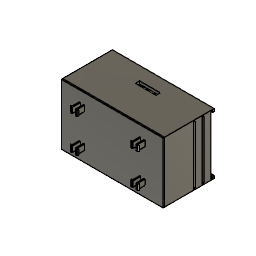
Control board - base v9 (Autodesk Fusion 360 design; units mm, degrees)
Autodesk Fusion 360 part; units mm, degrees
note: some values were not read from the file. Chosen so that the rebuilt part matches the saved one: which bodies a step acts on.
sketch "Esquisse1" plane through (0, 0, 0) normal (0, 1, 0) x (1, 0, 0)
  line L0 (-11.4317, -0.2961) -> (62.5683, -0.2961)
  line L1 (62.5683, -0.2961) -> (62.5683, -44.2961)
  line L2 (62.5683, -44.2961) -> (-11.4317, -44.2961)
  line L3 (-11.4317, -44.2961) -> (-11.4317, -0.2961)
  dimension "d1" = 74
  dimension "d2" = 44
  constraint horizontal L0
  constraint vertical L1
  constraint horizontal L2
  constraint vertical L3
  measures "d1" distance of L1 L3
  measures "d2" distance of L0 L2
extrude "Extrusion1" add sketch "Esquisse1" along normal blind 37.2 makes body 1
shell "Coque1" thickness 2 removed faces 1 at (37.9017, 37.2, 29.6294) on bodies 1
sketch "Sketch4" plane through (62.5683, 0, 0) normal (1, 0, 0) x (0, 1, 0)
  line L0 (0, 44.2961) -> (0, 0.2961)
  line L1 (0, 0.2961) -> (37.2, 0.2961)
  line L2 (37.2, 0.2961) -> (37.2, 44.2961)
  line L3 (37.2, 44.2961) -> (0, 44.2961)
  line L4 (0, 22.2961) -> (37.2, 22.2961) construction
  line L5 (22, 43.3961) -> (23.4, 43.3961)
  line L6 (23.4, 43.3961) -> (23.4, 1.1961)
  line L7 (23.4, 1.1961) -> (22, 1.1961)
  line L8 (22, 1.1961) -> (22, 43.3961)
  line L9 (29.8, 1.1961) -> (28.4, 1.1961)
  line L10 (28.4, 1.1961) -> (28.4, 43.3961)
  line L11 (28.4, 43.3961) -> (29.8, 43.3961)
  line L12 (29.8, 43.3961) -> (29.8, 1.1961)
  line L13 (34.8, 43.3961) -> (36.2, 43.3961)
  line L14 (36.2, 43.3961) -> (36.2, 1.1961)
  line L15 (36.2, 1.1961) -> (34.8, 1.1961)
  line L16 (34.8, 1.1961) -> (34.8, 43.3961)
  line L17 (36.2, 2.2961) -> (37.2, 2.2961)
  line L18 (37.2, 2.2961) -> (37.2, 42.2961)
  line L19 (37.2, 42.2961) -> (36.2, 42.2961)
  line L20 (36.2, 42.2961) -> (36.2, 2.2961)
  dimension "d16" = 42.2
  dimension "d17" = 42.2
  dimension "d18" = 42.2
  dimension "d19" = 1.4
  dimension "d20" = 1.4
  dimension "d21" = 1.4
  dimension "d54" = 22
  dimension "d55" = 5
  dimension "d56" = 5
  dimension "d57" = 40
  constraint midpoint L0 L4.start
  constraint midpoint L2 L4.end
  constraint horizontal L5
  constraint vertical L6
  constraint horizontal L7
  constraint vertical L8
  constraint symmetric L4 L5 L7
  constraint horizontal L9
  constraint vertical L10
  constraint horizontal L11
  constraint vertical L12
  constraint horizontal L13
  constraint vertical L14
  constraint horizontal L15
  constraint vertical L16
  constraint symmetric L4 L9 L11
  constraint symmetric L4 L13 L15
  constraint horizontal L17
  constraint vertical L18
  constraint horizontal L19
  constraint vertical L20
  constraint coincident L2 L18.end
  constraint coincident L14 L17.start
  constraint symmetric L4 L17 L19
  measures "d16" distance of L5.start L7.end
  measures "d17" distance of L9.end L10.end
  measures "d18" distance of L13.start L15.end
  measures "d19" distance of L6.end L7.end
  measures "d20" distance of L9.start L9.end
  measures "d21" distance of L14.end L15.end
  measures "d54" distance of L0 L8
  measures "d55" distance of L6 L10
  measures "d56" distance of L12 L16
  measures "d57" distance of L17.end L18.end
extrude "Extrude4" cut sketch "Sketch4" against normal blind 73.1 contours L13 L14 L15 L16 L20 | L5 L6 L7 L8 | L9 L10 L11 L12 bodies 1
ref_plane "WorkPlane1" through (25.5683, 18.6, 32.4961) normal (0, 0, 1) x (1, 0, 0)
sketch "Sketch5" plane through (0, 0, 32.4961) normal (0, 0, 1) x (1, 0, 0)
  line L0 (2.3683, 0) -> (2.3683, -5.74)
  line L1 (2.1083, -6) -> (1.3083, -6)
  line L2 (1.1018, -5.8979) -> (0.5683, -5.2)
  line L3 (0.5683, -5.2) -> (1.5683, -5.2)
  line L4 (1.5683, -5.2) -> (1.5683, 0)
  line L5 (1.5683, 0) -> (2.3683, 0)
  line L6 (62.5683, 0) -> (-11.4317, 0)
  arc A0 (2.1083, -6) -> (2.3683, -5.74) centre (2.1083, -5.74) ccw
  arc A1 (1.1018, -5.8979) -> (1.3083, -6) centre (1.3083, -5.74) ccw
  line L7 (-11.4317, 0) -> (-11.4317, 37.2)
  dimension "d26" = 6
  dimension "d27" = 5.2
  dimension "d28" = 0.26
  dimension "d29" = 0.8
  dimension "d30" = 0.8
  dimension "d31" = 1
  dimension "d47" = 13.8
  constraint vertical L0
  constraint perpendicular L0 L1
  constraint perpendicular L0 L3
  constraint perpendicular L3 L4
  constraint perpendicular L0 L5
  constraint tangent L0 A0
  constraint tangent L1 A0
  constraint tangent L1 A1
  constraint tangent L2 A1
  constraint equal A0 A1
  measures "d26" distance of L1 L5
  measures "d27" distance of L3 L6
  measures "d28" radius of A0
  measures "d29" distance of L1.start L1.end
  measures "d30" distance of L0.start L4.end
  measures "d31" distance of L2.end L3.end
  measures "d47" distance of L0 L7
sketch "Sketch7" plane through (0, 0, 32.4961) normal (0, 0, 1) x (1, 0, 0)
  line L0 (4.7683, 0) -> (5.5683, 0)
  line L1 (5.5683, 0) -> (5.5683, -5.2)
  line L2 (5.5683, -5.2) -> (6.5683, -5.2)
  line L3 (6.5683, -5.2) -> (6.0349, -5.8979)
  line L4 (5.8283, -6) -> (5.0283, -6)
  line L5 (4.7683, -5.74) -> (4.7683, 0)
  arc A0 (5.8283, -6) -> (6.0349, -5.8979) centre (5.8283, -5.74) ccw
  arc A1 (4.7683, -5.74) -> (5.0283, -6) centre (5.0283, -5.74) ccw
  line L6 (1.5683, -5.2) -> (1.5683, 0)
  dimension "d39" = 5.2
  dimension "d40" = 1
  dimension "d41" = 6
  dimension "d42" = 0.26
  dimension "d43" = 0.8
  dimension "d44" = 0.8
  dimension "d45" = 4
  constraint horizontal L0
  constraint perpendicular L0 L1
  constraint perpendicular L1 L2
  constraint parallel L2 L4
  constraint perpendicular L0 L5
  constraint tangent L3 A0
  constraint tangent L4 A0
  constraint tangent L4 A1
  constraint tangent L5 A1
  constraint equal A0 A1
  measures "d39" distance of L0.end L1.end
  measures "d40" distance of L1.end L2.end
  measures "d41" distance of L0 L4
  measures "d42" radius of A0
  measures "d43" distance of L4.start L4.end
  measures "d44" distance of L0.start L0.end
  measures "d45" distance of L1 L6
ref_plane "WorkPlane3" through (25.5683, 18.6, 22.2961) normal (-1, 0, 0) x (0, 0, 1)
ref_plane "WorkPlane4" through (25.5683, 18.6, 22.2961) normal (0, 0, 1) x (1, 0, 0)
extrude "Extrude5" add sketch "Sketch5" sketch "Sketch7" along normal blind 4 separate body of sketch 2 makes body 2 at (2.3683, -1.9133, 33.8294) makes body 3 at (4.7683, -3.8267, 33.8294)
mirror "Mirror1" about plane through (25.5683, 18.6, 22.2961) normal (-1, 0, 0) of bodies 2 3 makes body 4 at (48.7683, -1.9133, 33.8294) makes body 5 at (46.3683, -3.8267, 33.8294)
mirror "Mirror2" about plane through (25.5683, 18.6, 22.2961) normal (0, 0, 1) of bodies 2 3 5 4 makes body 6 at (2.3683, -1.9133, 10.7627) makes body 7 at (4.7683, -3.8267, 10.7627) makes body 8 at (48.7683, -1.9133, 10.7627) makes body 9 at (46.3683, -3.8267, 10.7627)
sketch "Sketch8" plane through (0, 37.2, 0) normal (0, 1, 0) x (-1, 0, 0)
  line L0 (9.4317, 42.2961) -> (9.4317, 2.2961)
  line L1 (9.4317, 2.2961) -> (-60.5683, 2.2961)
  line L2 (-60.5683, 2.2961) -> (-60.5683, 42.2961)
  line L3 (-60.5683, 42.2961) -> (9.4317, 42.2961)
  line L4 (11.4317, 44.2961) -> (-62.5683, 44.2961)
  line L5 (-62.5683, 44.2961) -> (-62.5683, 0.2961)
  line L6 (-62.5683, 0.2961) -> (11.4317, 0.2961)
  line L7 (11.4317, 0.2961) -> (11.4317, 44.2961)
  line L8 (-60.5683, 2.2961) -> (-62.5683, 2.2961)
  line L9 (-62.5683, 2.2961) -> (-62.5683, 42.2961)
  line L10 (-62.5683, 42.2961) -> (-60.5683, 42.2961)
  line L11 (-60.5683, 42.2961) -> (-60.5683, 2.2961)
  dimension "d58" = 40
  constraint horizontal L8
  constraint vertical L9
  constraint horizontal L10
  constraint vertical L11
  constraint coincident L1.end L2.start
  measures "d58" distance of L1.end L2.end
extrude "Extrude6" cut sketch "Sketch8" against normal blind 1 contours L2 L5 L8 L9 L10 L11 bodies 1
ref_plane "WorkPlane5" through (25.5683, 1, 22.2961) normal (0, 1, 0) x (1, 0, 0)
split "Split1" by plane through (25.5683, 1, 22.2961) normal (0, 1, 0) bodies 8 2 4 1 5 6 7 9 3 makes body 10 at (13.9017, 2, 28.9627)
combine "Combine1" operation add target body 1 tool bodies 2 3 4 5 6 7 8 9
sketch "Sketch9" plane through (0, 0, 44.2961) normal (0, 0, 1) x (-1, 0, 0)
  line L0 (11.4317, -1) -> (-62.5683, -1)
  line L1 (-62.5683, -1) -> (-62.5683, -37.2)
  line L2 (-62.5683, -37.2) -> (11.4317, -37.2)
  line L3 (11.4317, -37.2) -> (11.4317, -1)
  line L4 (-62.5683, -25.9) -> (11.4317, -25.9) construction
  line L5 (-33.0683, -24.4) -> (-18.0683, -24.4)
  line L6 (-18.0683, -24.4) -> (-18.0683, -27.4)
  line L7 (-18.0683, -27.4) -> (-33.0683, -27.4)
  line L8 (-33.0683, -27.4) -> (-33.0683, -24.4)
  line L9 (-25.5683, -37.2) -> (-25.5683, -1) construction
  dimension "d61" = 11.3
  dimension "d62" = 15
  dimension "d63" = 3
  constraint coincident L1 L4.start
  constraint coincident L3 L4.end
  constraint perpendicular L3 L4
  constraint horizontal L5
  constraint vertical L6
  constraint horizontal L7
  constraint vertical L8
  constraint symmetric L4 L5 L7
  constraint midpoint L2 L9.start
  constraint midpoint L0 L9.end
  constraint symmetric L6 L8 L9
  measures "d61" distance of L2 L4
  measures "d62" distance of L5.start L5.end
  measures "d63" distance of L5.end L6.end
extrude "Extrude7" cut sketch "Sketch9" against normal blind 51 contours L5 L6 L7 L8 bodies 10
